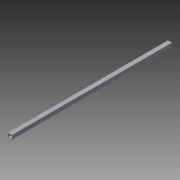
# Autodesk Inventor part: 40 inch extruded alluminum tube
Saved by Autodesk Inventor 2011 SP1 (Build 150282100, 282)
## iProperties
Created: 2011-01-11
Part Number: 40 inch extruded alluminum tube
Document SubType Name: Modeling
Designer: Christopher
Density: 1 g/cm^3
Author: Christopher
Autodesk Inventor part; units mm, degrees
ref_plane "YZ Plane" through (0, 0, 0) normal (1, 0, 0) x (0, 1, 0)
ref_plane "XZ Plane" through (0, 0, 0) normal (0, 1, 0) x (-1, 0, 0)
ref_plane "XY Plane" through (0, 0, 0) normal (0, 0, 1) x (1, 0, 0)
sketch "Sketch1" plane through (0, 0, 0) normal (0, 0, 1) x (1, 0, 0)
  line L0 (-13.0592, 7.1789) -> (12.3408, 7.1789)
  line L1 (12.3408, 7.1789) -> (12.3408, -18.2211)
  line L2 (12.3408, -18.2211) -> (-13.0592, -18.2211)
  line L3 (-13.0592, -18.2211) -> (-13.0592, 7.1789)
  line L4 (10.7533, 5.5914) -> (-11.4717, 5.5914)
  line L5 (-11.4717, 5.5914) -> (-11.4717, -16.6336)
  line L6 (-11.4717, -16.6336) -> (10.7533, -16.6336)
  line L7 (10.7533, -16.6336) -> (10.7533, 5.5914)
  point P0 (0, 0)
  dimension "d0" = 25.4
  dimension "d1" = 25.4
  dimension "d2" = 1.5875
  constraints: 16 end point, 4 parallel, 2 perpendicular, 1 horizontal, 3 other
  measures "d0" distance of L0.start L0.end
  measures "d1" distance of L2.end L0.start
  measures "d2" distance between parallel lines of L0 L4
extrude "Extrusion1" add sketch "Sketch1" against normal blind 1016
body "Solid1"
